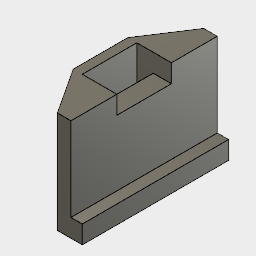
v1 Sensor Jig (Autodesk Fusion 360 design; units mm, degrees)
Autodesk Fusion 360 part; units mm, degrees
note: some values were not read from the file. Set by a fixed rule: which sketch regions a step uses.
sketch "Sketch1" plane through (0, 0, 0) normal (0, 1, 0) x (1, 0, 0)
  line L0 (10.55, -8.05) -> (-10.55, -8.05)
  line L1 (-10.55, -8.05) -> (-10.55, 8.05)
  line L2 (-10.55, 8.05) -> (10.55, 8.05)
  line L3 (10.55, 8.05) -> (10.55, -8.05)
  line L4 (10.55, -8.05) -> (-10.55, 8.05) construction
  line L5 (-10.55, -8.05) -> (10.55, 8.05) construction
  dimension "d1" = 21.1
  dimension "d2" = 16.1
  measures "d1" distance of L1.end L2.end
  measures "d2" distance of L0.end L1.end
extrude "Extrude1" add sketch "Sketch1" along normal blind 3.5 makes body 1
sketch "Sketch2" plane through (0, 3.5, 0) normal (0, 1, 0) x (-1, 0, 0)
  line L0 (-10.55, -8.05) -> (10.55, -8.05)
  line L1 (10.55, -8.05) -> (10.55, 8.05)
  line L2 (10.55, 8.05) -> (-10.55, 8.05)
  line L3 (-10.55, 8.05) -> (-10.55, -8.05)
  line L4 (-9.05, 6.55) -> (9.05, 6.55)
  line L5 (9.05, 6.55) -> (9.05, -6.55)
  line L6 (9.05, -6.55) -> (-9.05, -6.55)
  line L7 (-9.05, -6.55) -> (-9.05, 6.55)
  line L8 (-9.05, 6.55) -> (9.05, -6.55) construction
  line L9 (9.05, 6.55) -> (-9.05, -6.55) construction
  dimension "d5" = 18.1
  dimension "d6" = 13.1
  measures "d5" distance of L5.end L6.end
  measures "d6" distance of L4.end L5.end
extrude "Extrude2" cut sketch "Sketch2" against normal blind 1.5 contours L4 L5 L6 L7 bodies 1
extrude "Extrude3" add 1 faces at (-3.0167, 3.5, -7.55) along direction (0, 1, 0) blind 5.7 on bodies 1 bodies 1
sketch "Sketch3" plane through (0, 9.2, 0) normal (0, 1, 0) x (-1, 0, 0)
  line L0 (9.05, 6.55) -> (9.05, -6.55)
  line L1 (9.05, -6.55) -> (-9.05, -6.55)
  line L2 (-9.05, -6.55) -> (-9.05, 6.55)
  line L3 (-9.05, 6.55) -> (9.05, 6.55)
  line L4 (-10.55, -8.05) -> (10.55, -8.05)
  line L5 (10.55, -8.05) -> (10.55, 8.05)
  line L6 (10.55, 8.05) -> (-10.55, 8.05)
  line L7 (-10.55, 8.05) -> (-10.55, -8.05)
  line L8 (-9.05, -6.55) -> (-7.1, -6.55)
  line L9 (-7.1, -6.55) -> (-7.1, -8.05)
  line L10 (-7.1, -8.05) -> (-9.05, -8.05)
  line L11 (-9.05, -8.05) -> (-9.05, -6.55)
  line L12 (-7.1, -6.55) -> (-0.8, -6.55)
  line L13 (-0.8, -6.55) -> (-0.8, -8.05)
  line L14 (-0.8, -8.05) -> (-7.1, -8.05)
  line L15 (-7.1, -8.05) -> (-7.1, -6.55)
  dimension "d11" = 1.95
  dimension "d12" = 6.3
  measures "d11" distance of L1.end L8.end
  measures "d12" distance of L8.end L12.end
extrude "Extrude4" cut sketch "Sketch3" against normal blind 5.7 contours L1 L4 L9 L12 L13 L14 L15 bodies 1
sketch "Sketch4" plane through (0, 2, 0) normal (0, 1, 0) x (-1, 0, 0)
  line L0 (-9.05, -6.55) -> (9.05, -6.55)
  line L1 (9.05, -6.55) -> (9.05, 6.55)
  line L2 (9.05, 6.55) -> (-9.05, 6.55)
  line L3 (-9.05, 6.55) -> (-9.05, -6.55)
  line L4 (-0.8, -6.55) -> (-7.1, -6.55)
  line L5 (-7.1, -6.55) -> (-7.1, -8.05)
  line L6 (-7.1, -8.05) -> (-0.8, -8.05)
  line L7 (-0.8, -8.05) -> (-0.8, -6.55)
  line L8 (9.05, -6.55) -> (5.55, -6.55)
  line L9 (5.55, -6.55) -> (5.55, 6.55)
  line L10 (5.55, 6.55) -> (9.05, 6.55)
  line L11 (9.05, 6.55) -> (9.05, -6.55)
  dimension "d15" = 3.5
  measures "d15" distance of L0.end L8.end
extrude "Extrude5" cut sketch "Sketch4" against normal blind 1 contours L0 L1 L2 L8 L9 L10 L11 bodies 1
sketch "Sketch5" plane through (0, 9.2, 0) normal (0, 1, 0) x (-1, 0, 0)
  line L0 (-7.1, -8.05) -> (-7.1, -6.55)
  line L1 (-7.1, -6.55) -> (-9.05, -6.55)
  line L2 (-9.05, -6.55) -> (-9.05, 6.55)
  line L3 (-9.05, 6.55) -> (9.05, 6.55)
  line L4 (9.05, 6.55) -> (9.05, -6.55)
  line L5 (9.05, -6.55) -> (-0.8, -6.55)
  line L6 (-0.8, -6.55) -> (-0.8, -8.05)
  line L7 (-0.8, -8.05) -> (10.55, -8.05)
  line L8 (10.55, -8.05) -> (10.55, 8.05)
  line L9 (10.55, 8.05) -> (-10.55, 8.05)
  line L10 (-10.55, 8.05) -> (-10.55, -8.05)
  line L11 (-10.55, -8.05) -> (-7.1, -8.05)
  line L12 (12.85, -3) -> (8.25, -3)
  line L13 (8.25, -3) -> (8.25, 3)
  line L14 (8.25, 3) -> (12.85, 3)
  line L15 (12.85, 3) -> (12.85, -3)
  line L16 (12.85, -3) -> (8.25, 3) construction
  line L17 (8.25, -3) -> (12.85, 3) construction
  line L18 (12.85, -3) -> (13.85, -3)
  line L19 (13.85, -3) -> (13.85, 3)
  line L20 (13.85, 3) -> (12.85, 3)
  line L21 (12.85, 3) -> (12.85, -3)
  line L22 (10.55, -8.05) -> (10.55, 8.05)
  line L23 (10.55, 8.05) -> (13.85, 3)
  line L24 (13.85, -3) -> (10.55, -8.05)
  point P0 (10.55, 0)
  dimension "d18" = 4.6
  dimension "d19" = 6
  dimension "d20" = 1
  measures "d18" distance of L13.end L14.end
  measures "d19" distance of L12.end L13.end
  measures "d20" distance of L12.start L18.end
extrude "Extrude6" add sketch "Sketch5" against normal blind 9.2 contours L8 L14 L20 L22 L23 | L8 L12 L14 L15 L21 L22 | L15 L18 L19 L20 L21 | L8 L12 L18 L22 L24 bodies 1
sketch "Sketch6" plane through (0, 9.2, 0) normal (0, 1, 0) x (-1, 0, 0)
  line L0 (-7.1, -8.05) -> (-7.1, -6.55)
  line L1 (-7.1, -6.55) -> (-9.05, -6.55)
  line L2 (-9.05, -6.55) -> (-9.05, 6.55)
  line L3 (-9.05, 6.55) -> (9.05, 6.55)
  line L4 (9.05, 6.55) -> (9.05, -6.55)
  line L5 (9.05, -6.55) -> (-0.8, -6.55)
  line L6 (-0.8, -6.55) -> (-0.8, -8.05)
  line L7 (-0.8, -8.05) -> (10.55, -8.05)
  line L8 (10.55, -8.05) -> (13.85, -3)
  line L9 (13.85, -3) -> (13.85, 3)
  line L10 (13.85, 3) -> (10.55, 8.05)
  line L11 (10.55, 8.05) -> (-10.55, 8.05)
  line L12 (-10.55, 8.05) -> (-10.55, -8.05)
  line L13 (-10.55, -8.05) -> (-7.1, -8.05)
  line L14 (13.85, -3) -> (12.85, -3)
  line L15 (12.85, -3) -> (12.85, 3)
  line L16 (12.85, 3) -> (13.85, 3)
  line L17 (13.85, 3) -> (13.85, -3)
  line L18 (12.85, -3) -> (11.05, -3)
  line L19 (11.05, -3) -> (11.05, 3)
  line L20 (11.05, 3) -> (12.85, 3)
  line L21 (12.85, 3) -> (12.85, -3)
  dimension "d23" = 1
  dimension "d24" = 1.8
  measures "d23" distance of L8.end L14.end
  measures "d24" distance of L14.end L18.end
extrude "Extrude7" cut sketch "Sketch6" against normal blind 7.2 contours L15 L18 L19 L20 L21 bodies 1
extrude "Extrude8" add 1 faces at (-9.7167, 9.2, -1) along direction (0, 1, 0) blind 2 on bodies 1 bodies 1
sketch "Sketch7" plane through (0, 11.2, 0) normal (0, 1, 0) x (-1, 0, 0)
  line L0 (11.05, -3) -> (11.05, 3)
  line L1 (11.05, 3) -> (12.85, 3)
  line L2 (12.85, 3) -> (12.85, -3)
  line L3 (12.85, -3) -> (11.05, -3)
  line L4 (-7.1, -8.05) -> (-7.1, -6.55)
  line L5 (-7.1, -6.55) -> (-9.05, -6.55)
  line L6 (-9.05, -6.55) -> (-9.05, 6.55)
  line L7 (-9.05, 6.55) -> (9.05, 6.55)
  line L8 (9.05, 6.55) -> (9.05, -6.55)
  line L9 (9.05, -6.55) -> (-0.8, -6.55)
  line L10 (-0.8, -6.55) -> (-0.8, -8.05)
  line L11 (-0.8, -8.05) -> (10.55, -8.05)
  line L12 (10.55, -8.05) -> (13.85, -3)
  line L13 (13.85, -3) -> (13.85, 3)
  line L14 (13.85, 3) -> (10.55, 8.05)
  line L15 (10.55, 8.05) -> (-10.55, 8.05)
  line L16 (-10.55, 8.05) -> (-10.55, -8.05)
  line L17 (-10.55, -8.05) -> (-7.1, -8.05)
  line L18 (11.05, -3) -> (9.05, -3)
  line L19 (9.05, -3) -> (9.05, 3)
  line L20 (9.05, 3) -> (11.05, 3)
  line L21 (11.05, 3) -> (11.05, -3)
extrude "Extrude9" cut sketch "Sketch7" against normal blind 2 contours L0 L8 L18 L19 L20 L21 bodies 1
copy_body "Body->Comp1" bodies 1 removing the originals makes body 2 in component "WSSM-03: Lower Half "
sketch "Sketch1 (2)" plane through (0, 11.2, 0) normal (0, 1, 0) x (-1, 0, 0) in component "WSSM-04: Upper Half"
  line L0 (9.05, 3) -> (12.85, 3)
  line L1 (12.85, 3) -> (12.85, -3)
  line L2 (12.85, -3) -> (9.05, -3)
  line L3 (9.05, -3) -> (9.05, -6.55)
  line L4 (9.05, -6.55) -> (-0.8, -6.55)
  line L5 (-0.8, -6.55) -> (-0.8, -8.05)
  line L6 (-0.8, -8.05) -> (10.55, -8.05)
  line L7 (10.55, -8.05) -> (13.85, -3)
  line L8 (13.85, -3) -> (13.85, 3)
  line L9 (13.85, 3) -> (10.55, 8.05)
  line L10 (10.55, 8.05) -> (-10.55, 8.05)
  line L11 (-10.55, 8.05) -> (-10.55, -8.05)
  line L12 (-10.55, -8.05) -> (-7.1, -8.05)
  line L13 (-7.1, -8.05) -> (-7.1, -6.55)
  line L14 (-7.1, -6.55) -> (-9.05, -6.55)
  line L15 (-9.05, -6.55) -> (-9.05, 6.55)
  line L16 (-9.05, 6.55) -> (9.05, 6.55)
  line L17 (9.05, 6.55) -> (9.05, 3)
  line L18 (-9.05, 6.55) -> (-0.8, 6.55)
  line L19 (-0.8, 6.55) -> (-0.8, -6.55)
  line L20 (-0.8, -6.55) -> (-9.05, -6.55)
  line L21 (-9.05, -6.55) -> (-9.05, 6.55)
  line L22 (-0.8, -8.05) -> (-7.1, -8.05)
  line L23 (-7.1, -8.05) -> (-7.1, -6.55)
  line L24 (-7.1, -6.55) -> (-0.8, -6.55)
  line L25 (-0.8, -6.55) -> (-0.8, -8.05)
extrude "Extrude1'" add sketch "Sketch1 (2)" against normal blind 1.85 separate body contours L14 L15 L16 L18 L19 L20 L21 L24 | L5 L13 L20 L22 L23 L24 L25 makes body 3 in component "WSSM-04: Upper Half"
move_face "OffsetFaces1" offset -0.1 1 faces at (9.05, 10.5833, -2.1833) on bodies 3 in component "WSSM-04: Upper Half"
move_face "OffsetFaces2" offset -0.1 1 faces at (3.5167, 9.9667, 6.55) on bodies 3 in component "WSSM-04: Upper Half"
move_face "OffsetFaces3" offset -0.1 1 faces at (7.7167, 10.5833, -6.55) on bodies 3 in component "WSSM-04: Upper Half"
move_face "OffsetFaces4" offset -0.15 1 faces at (7.1, 10.5833, -7.5167) on bodies 3 in component "WSSM-04: Upper Half"
sketch "Sketch2 (2)" plane through (0, 11.2, 0) normal (0, 1, 0) x (-1, 0, 0) in component "WSSM-04: Upper Half"
  line L0 (9.05, 3) -> (12.85, 3)
  line L1 (12.85, 3) -> (12.85, -3)
  line L2 (12.85, -3) -> (9.05, -3)
  line L3 (9.05, -3) -> (9.05, -6.55)
  line L4 (9.05, -6.55) -> (-0.8, -6.55)
  line L5 (-0.8, -6.55) -> (-0.8, -8.05)
  line L6 (-0.8, -8.05) -> (10.55, -8.05)
  line L7 (10.55, -8.05) -> (13.85, -3)
  line L8 (13.85, -3) -> (13.85, 3)
  line L9 (13.85, 3) -> (10.55, 8.05)
  line L10 (10.55, 8.05) -> (-10.55, 8.05)
  line L11 (-10.55, 8.05) -> (-10.55, -8.05)
  line L12 (-10.55, -8.05) -> (-7.1, -8.05)
  line L13 (-7.1, -8.05) -> (-7.1, -6.55)
  line L14 (-7.1, -6.55) -> (-9.05, -6.55)
  line L15 (-9.05, -6.55) -> (-9.05, 6.55)
  line L16 (-9.05, 6.55) -> (9.05, 6.55)
  line L17 (9.05, 6.55) -> (9.05, 3)
  line L18 (9.05, -6.55) -> (-0.8, -6.55)
  line L19 (-0.8, -6.55) -> (-0.8, 6.45)
  line L20 (-0.8, 6.45) -> (9.05, 6.45)
  line L21 (9.05, 6.45) -> (9.05, -6.55)
  line L22 (9.05, -3) -> (12.85, -3)
  line L23 (12.85, -3) -> (12.85, 3)
  line L24 (12.85, 3) -> (9.05, 3)
  line L25 (9.05, 3) -> (9.05, -3)
  point P0 (-0.8, 6.45)
extrude "Extrude2'" add sketch "Sketch2 (2)" against normal blind 1 contours L3 L4 L17 L18 L19 L20 L21 L25 | L0 L1 L2 L21 L22 L23 L24 L25 bodies 3 in component "WSSM-04: Upper Half"
move_face "OffsetFaces5" offset -0.1 1 faces at (-9.05, 10.8667, 5.3) on bodies 3 in component "WSSM-04: Upper Half"
move_face "OffsetFaces6" offset -0.1 1 faces at (-10.25, 10.8667, 3) on bodies 3 in component "WSSM-04: Upper Half"
move_face "OffsetFaces7" offset -0.15 1 faces at (-12.85, 10.8667, 0.9333) on bodies 3 in component "WSSM-04: Upper Half"
move_face "OffsetFaces8" offset -0.1 1 faces at (-11.4833, 10.8667, -3) on bodies 3 in component "WSSM-04: Upper Half"
move_face "OffsetFaces9" offset -0.15 1 faces at (-9.05, 10.8667, -4.1167) on bodies 3 in component "WSSM-04: Upper Half"
move_face "OffsetFaces10" offset -0.1 1 faces at (-5.6667, 10.5333, -6.55) on bodies 3 in component "WSSM-04: Upper Half"
move_face "OffsetFaces11" offset -0.1 1 faces at (0.8, 10.25, -7.5167) on bodies 3 in component "WSSM-04: Upper Half"
sketch "Sketch3 (2)" plane through (0, 11.2, 0) normal (0, 1, 0) x (-1, 0, 0) in component "WSSM-04: Upper Half"
  line L0 (9.05, 3) -> (12.85, 3)
  line L1 (12.85, 3) -> (12.85, -3)
  line L2 (12.85, -3) -> (9.05, -3)
  line L3 (9.05, -3) -> (9.05, -6.55)
  line L4 (9.05, -6.55) -> (-0.8, -6.55)
  line L5 (-0.8, -6.55) -> (-0.8, -8.05)
  line L6 (-0.8, -8.05) -> (10.55, -8.05)
  line L7 (10.55, -8.05) -> (13.85, -3)
  line L8 (13.85, -3) -> (13.85, 3)
  line L9 (13.85, 3) -> (10.55, 8.05)
  line L10 (10.55, 8.05) -> (-10.55, 8.05)
  line L11 (-10.55, 8.05) -> (-10.55, -8.05)
  line L12 (-10.55, -8.05) -> (-7.1, -8.05)
  line L13 (-7.1, -8.05) -> (-7.1, -6.55)
  line L14 (-7.1, -6.55) -> (-9.05, -6.55)
  line L15 (-9.05, -6.55) -> (-9.05, 6.55)
  line L16 (-9.05, 6.55) -> (9.05, 6.55)
  line L17 (9.05, 6.55) -> (9.05, 3)
  line L18 (-10.55, -8.05) -> (10.55, -8.05)
  line L19 (13.85, -3) -> (13.85, 3)
  line L20 (10.55, 8.05) -> (-10.55, 8.05)
extrude "Extrude3'" add sketch "Sketch3 (2)" along normal blind 2 bodies 3 in component "WSSM-04: Upper Half"
sketch "Sketch4 (2)" plane through (-13.85, 0, 0) normal (-1, 0, 0) x (0, 0, 1) in component "WSSM-04: Upper Half"
  line L0 (-3, 11.2) -> (3, 11.2)
  line L1 (3, 11.2) -> (3, 13.2)
  line L2 (3, 13.2) -> (-3, 13.2)
  line L3 (-3, 13.2) -> (-3, 11.2)
  line L4 (-3, 11.2) -> (3, 11.2)
  line L5 (3, 11.2) -> (3, 12.2)
  line L6 (3, 12.2) -> (-3, 12.2)
  line L7 (-3, 12.2) -> (-3, 11.2)
extrude "Extrude4'" cut sketch "Sketch4 (2)" against normal blind 1 contours L0 L1 L3 L4 L5 L6 L7 bodies 3 in component "WSSM-04: Upper Half"
sketch "Sketch5 (2)" plane through (10.55, 0, 0) normal (1, 0, 0) x (0, 0, -1) in component "WSSM-04: Upper Half"
  line L0 (-8.05, 11.2) -> (8.05, 11.2)
  line L1 (8.05, 11.2) -> (8.05, 13.2)
  line L2 (8.05, 13.2) -> (-8.05, 13.2)
  line L3 (-8.05, 13.2) -> (-8.05, 11.2)
  line L4 (3, 12.2) -> (-3, 12.2)
  line L5 (-3, 12.2) -> (-3, 10.2)
  line L6 (-3, 10.2) -> (3, 10.2)
  line L7 (3, 10.2) -> (3, 12.2)
  line L8 (3, 12.2) -> (-3, 10.2) construction
  line L9 (-3, 12.2) -> (3, 10.2) construction
  line L10 (-3, 12.2) -> (3, 12.2)
  line L11 (3, 12.2) -> (3, 11.2)
  line L12 (3, 11.2) -> (-3, 11.2)
  line L13 (-3, 11.2) -> (-3, 12.2)
  point P0 (0, 11.2)
  dimension "d50" = 6
  dimension "d51" = 2
  dimension "d52" = 6
  dimension "d53" = 1
  measures "d50" distance of L5.end L6.end
  measures "d51" distance of L4.end L5.end
  measures "d52" distance of L4.end L4.start
  measures "d53" distance of L4.end L12.end
extrude "Extrude5'" cut sketch "Sketch5 (2)" against normal blind 1 contours L0 L4 L5 L7 L10 L11 L12 L13 bodies 3 in component "WSSM-04: Upper Half"
sketch "Sketch8" plane through (-9.05, 0, 0) normal (1, 0, 0) x (0, 0, -1)
  line L0 (-3, 9.2) -> (-3, 11.2)
  line L1 (-3, 11.2) -> (-6.55, 11.2)
  line L2 (-6.55, 11.2) -> (-6.55, 1)
  line L3 (-6.55, 1) -> (6.55, 1)
  line L4 (6.55, 1) -> (6.55, 11.2)
  line L5 (6.55, 11.2) -> (3, 11.2)
  line L6 (3, 11.2) -> (3, 9.2)
  line L7 (3, 9.2) -> (-3, 9.2)
  line L8 (-9, 13) -> (9.4138, 13)
  line L9 (9.4138, 13) -> (9.4138, -1)
  line L10 (9.4138, -1) -> (-9, -1)
  line L11 (-9, -1) -> (-9, 13)
extrude "Extrude1''" cut sketch "Sketch8" along normal through all contours L0 L1 L2 L3 L4 L5 L6 L7 | L8 L9 L10 L11 bodies 2 in component "WSSM-03: Lower Half "
sketch "Sketch9" plane through (-13.85, 0, 0) normal (-1, 0, 0) x (0, 0, 1)
  line L0 (-3, 11.2) -> (-3, 0)
  line L1 (-3, 0) -> (3, 0)
  line L2 (3, 0) -> (3, 11.2)
  line L3 (3, 11.2) -> (-3, 11.2)
  line L4 (1.7549, 6.6) -> (-1.7451, 6.6)
  line L5 (-1.7451, 6.6) -> (-1.7451, 4.6)
  line L6 (-1.7451, 4.6) -> (1.7549, 4.6)
  line L7 (1.7549, 4.6) -> (1.7549, 6.6)
  line L8 (1.7549, 6.6) -> (-1.7451, 4.6) construction
  line L9 (-1.7451, 6.6) -> (1.7549, 4.6) construction
  point P0 (0.0049, 5.6)
  dimension "d57" = 3.5
  dimension "d58" = 2
  measures "d57" distance of L5.end L6.end
  measures "d58" distance of L4.end L5.end
extrude "Extrude2''" cut sketch "Sketch9" against normal blind 1 contours L4 L5 L6 L7 bodies 2 in component "WSSM-03: Lower Half "
sketch "Sketch10" plane through (-9.05, 0, 0) normal (1, 0, 0) x (0, 0, -1)
  line L0 (-3, 9.2) -> (-3, 11.2)
  line L1 (-3, 11.2) -> (-8.05, 11.2)
  line L2 (-8.05, 11.2) -> (-8.05, 0)
  line L3 (-8.05, 0) -> (8.05, 0)
  line L4 (8.05, 0) -> (8.05, 11.2)
  line L5 (8.05, 11.2) -> (3, 11.2)
  line L6 (3, 11.2) -> (3, 9.2)
  line L7 (3, 9.2) -> (-3, 9.2)
  line L8 (8.05, 11.2) -> (8.05, 2)
  line L9 (8.05, 2) -> (-8.05, 2)
  line L10 (-8.05, 2) -> (-8.05, 0)
  line L11 (-8.05, 0) -> (8.05, 0)
  line L12 (8.05, 0) -> (8.05, 2)
  dimension "d61" = 9.2
  measures "d61" distance of L4.end L8.end
extrude "Extrude3''" add sketch "Sketch10" along normal blind 1.25 contours L2 L3 L4 L9 L10 L11 L12 bodies 2 in component "WSSM-03: Lower Half "
component "WSSM-03: Lower Half " placed x (1, 0, 0) y (0, 1, 0) z (0, 0, 1) at (0, 0, 0)
component "WSSM-04: Upper Half" placed x (1, 0, 0) y (0, 1, 0) z (0, 0, 1) at (0, 0, 0)
